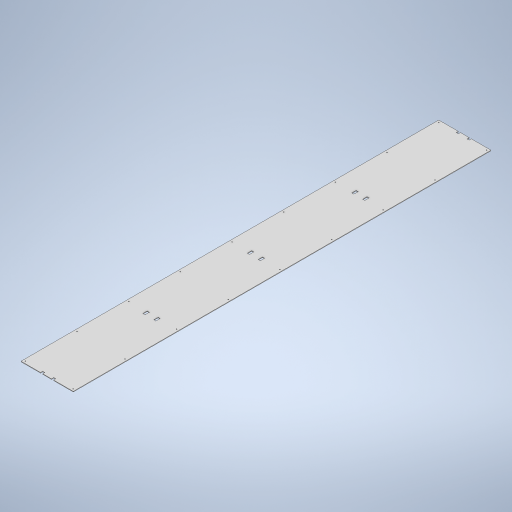
# Autodesk Inventor part: Plate1ftx8ft
Saved by Autodesk Inventor 2023 (Build 270158030, 158C)
## iProperties
Created: 2023-02-13
Part Number: Plate1ftx8ft
Material: Generic
Document SubType Name: Modeling
Designer: jeremyy
Density: 1 g/cm^3
Appearance: Default
Author: jeremyy
Autodesk Inventor part; units mm, degrees
ref_plane "YZ Plane" through (0, 0, 0) normal (1, 0, 0) x (0, 1, 0)
ref_plane "XZ Plane" through (0, 0, 0) normal (0, 1, 0) x (-1, 0, 0)
ref_plane "XY Plane" through (0, 0, 0) normal (0, 0, 1) x (1, 0, 0)
sketch "Sketch1" plane through (0, 0, 0) normal (0, 1, 0) x (-1, 0, 0)
  line L0 (0, 0) -> (304.8, 0)
  line L1 (304.8, 0) -> (304.8, -2438.4)
  line L2 (304.8, -2438.4) -> (0, -2438.4)
  line L3 (0, -2438.4) -> (0, 0)
  line L4 (114.3, 0) -> (127, 0)
  line L5 (127, 0) -> (127, -12.7)
  line L6 (127, -12.7) -> (114.3, -12.7)
  line L7 (114.3, -12.7) -> (114.3, 0)
  line L8 (152.4, -2438.4) -> (152.4, -2413)
  line L9 (127, -1219.2) -> (114.3, -1219.2)
  line L10 (114.3, -1219.2) -> (114.3, -1206.5)
  line L11 (114.3, -1206.5) -> (127, -1206.5)
  line L12 (127, -1206.5) -> (127, -1219.2)
  line L13 (114.3, -2438.4) -> (127, -2438.4)
  line L14 (127, -2438.4) -> (127, -2425.7)
  line L15 (127, -2425.7) -> (114.3, -2425.7)
  line L16 (114.3, -2425.7) -> (114.3, -2438.4)
  line L17 (114.3, -1219.2) -> (114.3, -1231.9)
  line L18 (114.3, -1231.9) -> (127, -1231.9)
  line L19 (127, -1231.9) -> (127, -1219.2)
  line L20 (190.5, 0) -> (177.8, 0)
  line L21 (177.8, 0) -> (177.8, -12.7)
  line L22 (177.8, -12.7) -> (190.5, -12.7)
  line L23 (190.5, -12.7) -> (190.5, 0)
  line L24 (177.8, -1219.2) -> (190.5, -1219.2)
  line L25 (190.5, -1219.2) -> (190.5, -1206.5)
  line L26 (190.5, -1206.5) -> (177.8, -1206.5)
  line L27 (177.8, -1206.5) -> (177.8, -1219.2)
  line L28 (190.5, -1231.9) -> (177.8, -1231.9)
  line L29 (190.5, -1219.2) -> (190.5, -1231.9)
  line L30 (177.8, -1231.9) -> (177.8, -1219.2)
  line L31 (177.8, -2425.7) -> (190.5, -2425.7)
  line L32 (190.5, -2438.4) -> (177.8, -2438.4)
  line L33 (177.8, -2438.4) -> (177.8, -2425.7)
  line L34 (190.5, -2425.7) -> (190.5, -2438.4)
  line L35 (127, -596.9) -> (114.3, -596.9)
  line L36 (114.3, -596.9) -> (114.3, -622.3)
  line L37 (114.3, -622.3) -> (127, -622.3)
  line L38 (127, -622.3) -> (127, -596.9)
  line L39 (127, -1841.5) -> (114.3, -1841.5)
  line L40 (114.3, -1841.5) -> (114.3, -1816.1)
  line L41 (114.3, -1816.1) -> (127, -1816.1)
  line L42 (127, -1816.1) -> (127, -1841.5)
  line L43 (177.8, -596.9) -> (190.5, -596.9)
  line L44 (190.5, -596.9) -> (190.5, -622.3)
  line L45 (190.5, -622.3) -> (177.8, -622.3)
  line L46 (177.8, -622.3) -> (177.8, -596.9)
  line L47 (177.8, -1841.5) -> (190.5, -1841.5)
  line L48 (177.8, -1816.1) -> (177.8, -1841.5)
  line L49 (190.5, -1816.1) -> (177.8, -1816.1)
  line L50 (190.5, -1841.5) -> (190.5, -1816.1)
  circle A0 centre (292.1, -12.7) radius 2.3812
  circle A1 centre (292.1, -314.325) radius 2.3813
  circle A2 centre (292.1, -615.95) radius 2.3813
  line L51 (304.8, -615.95) -> (300.4096, -615.95)
  circle A3 centre (292.1, -1219.2) radius 2.3812
  circle A4 centre (292.1, -917.575) radius 2.3813
  circle A5 centre (292.1, -2425.7) radius 2.3812
  circle A6 centre (292.1, -1822.45) radius 2.3813
  circle A7 centre (292.1, -1520.825) radius 2.3813
  circle A8 centre (292.1, -2124.075) radius 2.3813
  circle A9 centre (12.7, -12.7) radius 2.3812
  circle A10 centre (12.7, -314.325) radius 2.3813
  circle A11 centre (12.7, -615.95) radius 2.3813
  circle A12 centre (12.7, -1219.2) radius 2.3812
  circle A13 centre (12.7, -917.575) radius 2.3813
  circle A14 centre (12.7, -1520.825) radius 2.3813
  circle A15 centre (12.7, -1822.45) radius 2.3813
  circle A16 centre (12.7, -2425.7) radius 2.3812
  circle A17 centre (12.7, -2124.075) radius 2.3813
  point P0 (190.5, 0)
  point P1 (127, 0)
  point P2 (114.3, -2438.4)
  point P3 (127, -2438.4)
  dimension "d0" = 304.8
  dimension "d1" = 2438.4
  dimension "d4" = 12.7
  dimension "d5" = 12.7
  dimension "d6" = 114.3
  dimension "d7" = 25.4
  dimension "d8" = 12.7
  dimension "d9" = 12.7
  dimension "d10" = 114.3
  dimension "d11" = 1219.2
  dimension "d12" = 12.7
  dimension "d13" = 25.4
  dimension "d14" = 114.3
  dimension "d15" = 596.9
  dimension "d16" = 4.7625
  dimension "d17" = 12.7
  dimension "d18" = 12.7
  dimension "d19" = 4.7625
  dimension "d20" = 314.325
  dimension "d21" = 0
  dimension "d22" = 4.7625
  dimension "d23" = 0
  dimension "d24" = 615.95
  constraints: 104 end point, 47 symmetric about line, 18 centre point, 8 parallel, 5 horizontal, 4 perpendicular, 2 point on line, 1 midpoint, 1 vertical, 15 other
  measures "d0" distance of L1.end L2.end
  measures "d1" distance of L0.end L1.end
  measures "d4" distance of L5.end L6.end
  measures "d5" distance of L4.end L5.end
  measures "d6" distance between parallel lines of L3 L7
  measures "d7" distance of L8.start L8.end
  measures "d8" distance of L10.end L11.end
  measures "d9" distance of L9.end L10.end
  measures "d10" distance between parallel lines of L3 L10
  measures "d11" distance between parallel lines of L0 L9
  measures "d12" distance of L37.end L36.end
  measures "d13" distance of L36.end L35.end
  measures "d14" distance between parallel lines of L3 L36
  measures "d15" distance between parallel lines of L0 L35
  measures "d16" diameter of A0
  measures "d17" distance from line of L0 A0.centre
  measures "d18" distance from line of L1 A0.centre
  measures "d19" diameter of A1
  measures "d20" distance from line of L0 A1.centre
  measures "d21" horizontal distance of A0.centre A1.centre
  measures "d22" diameter of A2
  measures "d23" horizontal distance of A1.centre A2.centre
  measures "d24" distance from line of L0 A2.centre
extrude "Extrusion1" add sketch "Sketch1" along normal blind 3.175 contours L0 L7 L6 L5 L21 L22 L23 L1 L2 L34 L31 L33 L14 L15 L16 L3
body "Solid1"
